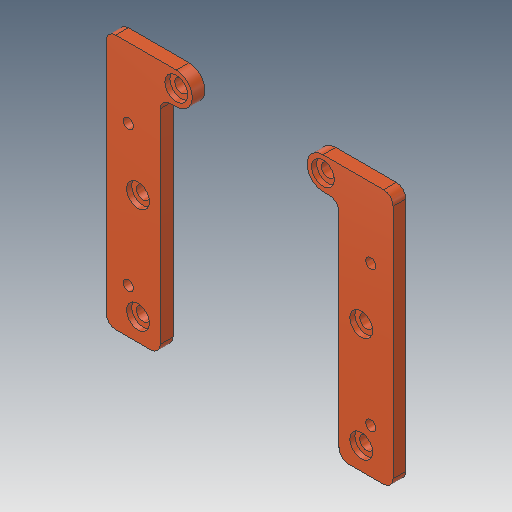
# Autodesk Inventor part: battery_cover_base
Saved by Autodesk Inventor 2019.4 (Build 234330000, 330)
## iProperties
Created: 2018-08-19
Part Number: battery_cover_base
Material: 一般
Document SubType Name: Modeling
Designer: y6tada
Density: 1 g/cm^3
Appearance: 滑らか - 淡いオレンジ
Mass: 1.35553 g
Surface Area: 19.3887 cm^2
Volume: 1.35553 cm^3
Author: y6tada
Autodesk Inventor part; units mm, degrees
ref_plane "YZ Plane" through (0, 0, 0) normal (1, 0, 0) x (0, 1, 0)
ref_plane "XZ Plane" through (0, 0, 0) normal (0, 1, 0) x (-1, 0, 0)
ref_plane "XY Plane" through (0, 0, 0) normal (0, 0, 1) x (1, 0, 0)
sketch "スケッチ1" plane through (0, 0, 0) normal (0, 0, 1) x (1, 0, 0)
  line L0 (0, 2.2573) -> (0, 51.1276) construction
  line L1 (22.5, 18.5) -> (22.5, -18.5)
  line L2 (19, 9) -> (19, 13) construction
  line L3 (19, -9) -> (19, -13) construction
  line L4 (14, 13.5) -> (14, -18.5)
  line L5 (11.5, 20) -> (21, 20)
  circle A0 centre (17.5, 0) radius 1.05
  circle A1 centre (11.5, 17.5) radius 1.05
  line L6 (17.5, 0) -> (17.5, -16.5) construction
  circle A2 centre (17.5, -16.5) radius 1.05
  arc A3 (11.5, 20) -> (11.5, 15) centre (11.5, 17.5) ccw
  line L7 (15.5, -20) -> (21, -20)
  arc A4 (21, -20) -> (22.5, -18.5) centre (21, -18.5) ccw
  arc A5 (22.5, 18.5) -> (21, 20) centre (21, 18.5) ccw
  arc A6 (14, -18.5) -> (15.5, -20) centre (15.5, -18.5) ccw
  line L8 (-4.5621, 0) -> (27.3728, 0) construction
  line L9 (11.5, 15) -> (12.5, 15)
  arc A7 (14, 13.5) -> (12.5, 15) centre (12.5, 13.5) ccw
  circle A8 centre (19, 9) radius 0.8
  circle A9 centre (19, -13) radius 0.8
  dimension "d6" = 4
  dimension "d10" = 4
  dimension "d19" = 2.1
  dimension "d20" = 9
  dimension "d22" = 2.1
  dimension "d28" = 38
  dimension "d29" = 45
  dimension "d41" = 3.5
  dimension "d46" = 2.5
  dimension "d47" = 35
  dimension "d48" = 9
  dimension "d50" = 22
  dimension "d51" = 1.5
  dimension "d52" = 3.5
  dimension "d53" = 1.5
  dimension "d54" = 40
  dimension "d55" = 28
  dimension "d56" = 1.5
  dimension "d57" = 2.5
  dimension "d58" = 1.6
  dimension "d59" = 1.6
  constraints: 18 end point, 10 centre point, 10 point on circle, 10 tangent, 7 vertical, 3 coincident, 3 horizontal, 2 equal radius, 1 collinear, 1 concentric, 1 other
  measures "d6" distance of L2.start L2.end
  measures "d10" distance of L3.start L3.end
  measures "d19" diameter of A0
  measures "d20" vertical distance of L6.start L2.start
  measures "d22" diameter of A1
  measures "d28" diameter of L2 L0
  measures "d29" diameter of L1 L0
  measures "d41" vertical distance of L3.end L6.end
  measures "d46" radius of A3
  measures "d47" diameter of L6 L0
  measures "d48" vertical distance of L3.start L6.start
  measures "d50" distance of L3.start L2.end
  measures "d51" radius of A4
  measures "d52" distance from line of L7 A2.centre
  measures "d53" radius of A6
  measures "d54" distance between parallel lines of L7 L5
  measures "d55" diameter of L4 L0
  measures "d56" radius of A7
  measures "d57" distance from line of L4 A1.centre
  measures "d58" diameter of A8
  measures "d59" diameter of A9
extrude "押し出し1" add sketch "スケッチ1" along normal blind 2
sketch "スケッチ3" plane through (0, 0, 2) normal (0, 0, 1) x (1, 0, 0)
  circle A0 centre (17.5, 0) radius 1.05 projected
  circle A1 centre (17.5, 0) radius 1.8
  circle A2 centre (11.5, 17.5) radius 1.05 projected
  circle A3 centre (11.5, 17.5) radius 1.8
  circle A4 centre (17.5, -16.5) radius 1.05 projected
  circle A5 centre (17.5, -16.5) radius 1.8
  point P0 (0, 0)
  dimension "d33" = 3.6
  constraints: 3 centre point, 3 coincident, 2 equal radius
  measures "d33" diameter of A3
extrude "押し出し2" cut sketch "スケッチ3" against normal blind 0.8
mirror "ミラー1" about plane through (0, 0, 0) normal (1, 0, 0) of "押し出し1", "押し出し2"
